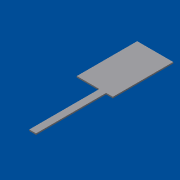
# Autodesk Inventor part: Tampa de trás 10-06-2016
Saved by Autodesk Inventor 2015 (Build 190159000, 159)
## iProperties
Created: 2016-06-10
Part Number: Tampa de trás 10-06-2016
Material: Genérico
Document SubType Name: Modeling
Designer: kelliton
Density: 1 g/cm^3
Appearance: Padrão
Author: kelliton
Autodesk Inventor part; units mm, degrees
ref_plane "YZ Plane" through (0, 0, 0) normal (1, 0, 0) x (0, 1, 0)
ref_plane "XZ Plane" through (0, 0, 0) normal (0, 1, 0) x (-1, 0, 0)
ref_plane "XY Plane" through (0, 0, 0) normal (0, 0, 1) x (1, 0, 0)
sketch "Esboço1" plane through (0, 0, 0) normal (0, 0, 1) x (1, 0, 0)
  line L0 (-37.1093, 20.0517) -> (-10.6595, 20.0517)
  line L1 (-10.6595, 20.0517) -> (-37.1093, 20.0517)
  line L2 (-10.6595, 20.0517) -> (-10.6595, -24.2254)
  line L3 (-10.6595, -24.2254) -> (-15.5932, -24.2254)
  line L4 (-15.5932, -24.2254) -> (-15.5932, -75.6194)
  line L5 (-15.5932, -24.2254) -> (-15.5932, -75.6194)
  line L6 (-15.5932, -75.6194) -> (-20.5932, -75.6194)
  line L7 (-20.5932, -75.6194) -> (-20.5932, -24.2254)
  line L8 (-20.5932, -75.6194) -> (-20.5932, -24.2254)
  line L9 (-20.5932, -24.2254) -> (-37.1093, -24.2254)
  line L10 (-20.5932, -24.2254) -> (-37.1093, -24.2254)
  line L11 (-37.1093, -24.2254) -> (-37.1093, 20.0517)
  point P0 (0, 0)
  point P1 (0, 0)
  constraints: 24 end point, 4 collinear, 4 perpendicular
extrude "Extrusão1" add sketch "Esboço1" along normal blind 1
